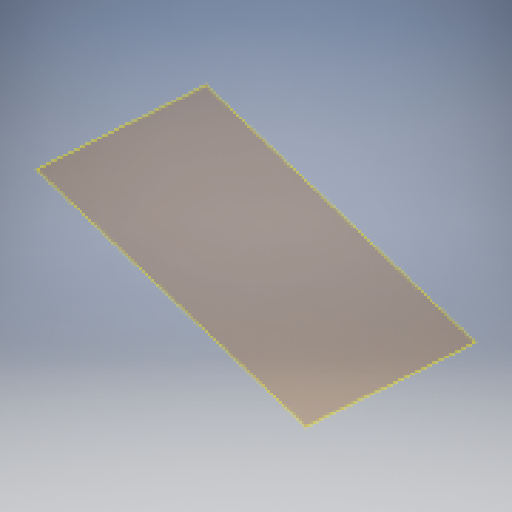
# Autodesk Inventor part: CE-5.2.3-02
Saved by Autodesk Inventor 2024 (Build 280153000, 153)
## iProperties
Created: 2024-02-15
Part Number: CE-5.2.3-02
Material: Generic
Document SubType Name: Sheet Metal
Designer: Alex
Density: 1 g/cm^3
Sheet Metal Rule: Default
Appearance: Default
Author: Alex
Autodesk Inventor part; units mm, degrees
ref_plane "YZ Plane" through (0, 0, 0) normal (1, 0, 0) x (0, 1, 0)
ref_plane "XZ Plane" through (0, 0, 0) normal (0, 1, 0) x (-1, 0, 0)
ref_plane "XY Plane" through (0, 0, 0) normal (0, 0, 1) x (1, 0, 0)
ref_plane "Work Plane1" through (660.1765, -750.8185, -321.5593) normal (0.2347344, 0.9720596, 0) x (0.9701425, -0.2342714, 0.0627728)
ref_plane "Work Plane2" through (660.1765, -750.8185, -1239.1973) normal (-0.2347344, -0.9720596, 0) x (0.9701425, -0.2342714, -0.0627728)
sketch "Sketch1" plane through (660.1765, -750.8185, -1239.1973) normal (-0.2347344, -0.9720596, 0) x (0.9701425, -0.2342714, -0.0627728)
  line L0 (1695.5374, 1112.9167) -> (113.5836, 913.1264) construction
  line L1 (217.7912, 25.13) -> (161.6208, 918.1852) construction
  line L2 (1764.0187, 24.13) -> (169.4987, 24.13) construction
  line L3 (1647.626, 1105.8579) -> (1715.6004, 25.13) construction
  line L4 (1647.5631, 1106.8579) -> (1715.6633, 24.13)
  line L5 (161.5579, 919.1852) -> (217.8541, 24.13)
  line L6 (217.8541, 24.13) -> (1715.6633, 24.13)
  line L7 (161.5579, 919.1852) -> (1647.5631, 1106.8579)
  point P0 (-894.1485, 1185.4069)
extrude "Plate1" add sketch "Sketch1" along normal blind 3.048
equation "\"d0\" = Thickness"
equation "\"BendRadius\" = Thickness"
equation "\"BendReliefWidth\" = Thickness"
equation "\"BendReliefDepth\" = 0.5 * Thickness"
equation "\"CornerReliefSize\" = 4 * Thickness"
equation "\"MinimumRemnant\" = 2 * Thickness"
equation "\"TransitionRadius\" = BendRadius"
equation "\"JacobiRadiusSize\" = BendRadius"
equation "\"GapSize\" = Thickness"
equation "\"Thickness\" = 3.048"
body "Solid1"
